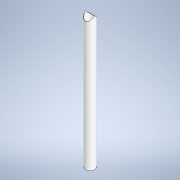
# Autodesk Inventor part: SP12V1 Agarre Baranda
Saved by Autodesk Inventor 2021.2 (Build 252289000, 289)
## iProperties
Created: 2026-05-26
Part Number: SP12V1 Agarre Baranda
Material: Acero, carbono
Document SubType Name: Modeling
Designer: nelso
Density: 7.85 g/cm^3
Appearance: Blanco
Author: nelso
Autodesk Inventor part; units mm, degrees
ref_plane "YZ Plane" through (0, 0, 0) normal (1, 0, 0) x (0, 1, 0)
ref_plane "XZ Plane" through (0, 0, 0) normal (0, 1, 0) x (-1, 0, 0)
ref_plane "XY Plane" through (0, 0, 0) normal (0, 0, 1) x (1, 0, 0)
sketch "Sketch1" plane through (0, 0, 0) normal (0, 1, 0) x (-1, 0, 0)
  circle A0 centre (0, 0) radius 15.55
  circle A1 centre (0, 0) radius 14.75
  dimension "d0" = 31.1
  dimension "d1" = 29.5
  constraints: 2 centre point, 2 coincident
  measures "d0" diameter of A0
  measures "d1" diameter of A1
extrude "Extrusion1" add sketch "Sketch1" along normal mid plane 445
sketch "Sketch6" plane through (0, 0, 0) normal (0, 0, 1) x (1, 0, 0)
  circle A0 centre (0, 222.5) radius 15.55 projected
  point P0 (0, 0)
extrude "Extrusion6" cut sketch "Sketch6" along normal mid plane 200
body "Solid1"
